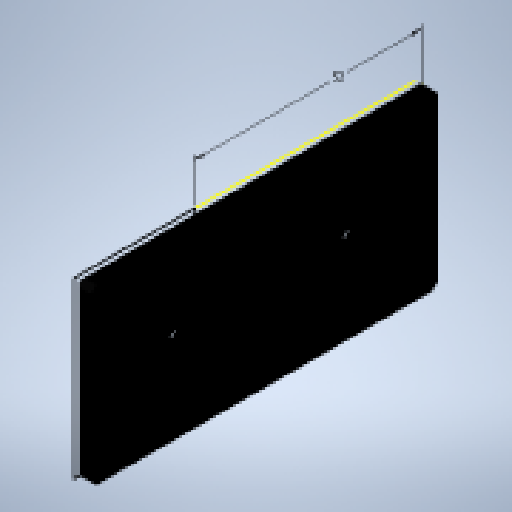
# Autodesk Inventor part: Robotunits CAP_4080_1
Saved by Autodesk Inventor 2023 (Build 270158000, 158)
## iProperties
Category: PARTsolutions
Company: ROBOTUNITS
Created: 2023-08-22
Part Number: Robotunits CAP_4080_1
Material: ABS PlastiK
Catalog Web Link: www.cadenas.de
Description: CAP_1-End Cap
Vendor: ROBOTUNITS
Document SubType Name: Modeling
Designer: psAdmin
Manufacturer: ROBOTUNITS
Mass: 13.3863 g
Surface Area: 73.9102 cm^2
Volume: 12.6286 cm^3
Density: 1.06 g/cm^3
Appearance: Generic
PSOL_IDENT_0: {$CADENAS_DATA/23d-libs/robotunits/pool_bauteile/cap.prj},182 {VTYP=3D},{NB=Robotunits CAP_4080_1},{
PSOL_IDENT_1: LINA=Robotunits CAP_4080_1},{NN=CAP_1},{DATE=24.04.2023 05:54:15},{GEOMDATE=22.02.2023 09:25:00},{VE
PSOL_IDENT_2: RSION=},{LINEID=120},{WBVAR=},{WBNUMERIC=}  {NB=Robotunits CAP_4080_1},{LINA=Robotunits CAP_4080_1},
PSOL_IDENT_3: {KT=DUMMY},{ARTIKEL=CAP_4080},{L=40},{B=80},{H=4},{GEW=0.009},{INFO=INFO},{V=2.000}
NB: Robotunits CAP_4080_1
NN: CAP_1
NT: End Cap
NBSYN: Robotunits $ARTIKEL._1
LINA: Robotunits CAP_4080_1
CATALOG: Robotunits
ARTIKEL: CAP_4080
L: 40
B: 80
H: 4
GEW: 0.009
INFO: INFO
SUPPLIER: ROBOTUNITS
ARTICLENO: Robotunits CAP_4080_1
BOMINFO: Robotunits CAP_4080_1
CREATOR: CADENAS GmbH
Title: Robotunits CAP_4080_1
Author: Cadenas PARTsolutions
Comments: End Cap
Autodesk Inventor part; units mm, degrees
sketch "Skizze_1" plane through (0, 0, 0) normal (1, 0, 0) x (0, 0, -1)
  line L0 (-40, 20) -> (-40, -20)
  line L1 (-40, -20) -> (40, -20)
  line L2 (40, -20) -> (40, 20)
  line L3 (40, 20) -> (-40, 20)
  constraints: 8 end point
extrude "Extrusion1" add sketch "Skizze_1" along normal blind 4
sketch "Sketch2" plane through (0, 0, 0) normal (-1, 0, 0) x (0, 0, 1)
  point P0 (20, 0)
hole "Hole1" at (0, 0, 20) direction (1, 0, 0) diameter 4 depth 4 countersink diameter 8.1 countersink angle 90
sketch "Sketch3" plane through (0, 0, 0) normal (-1, 0, 0) x (0, 0, 1)
  point P0 (-20, 0)
hole "Hole2" at (0, 0, -20) direction (1, 0, 0) diameter 4 depth 4 countersink diameter 8.1 countersink angle 90
ref_plane "CS_ANBAU_CAP_XY" through (0, 0, 0) normal (0, 1, 0) x (1, 0, 0)
ref_plane "CS_ANBAU_CAP_YZ" through (0, 0, 0) normal (1, 0, 0) x (0, 0, -1)
ref_plane "CS_ANBAU_CAP_ZX" through (0, 0, 0) normal (0, 0, -1) x (0, 1, 0)
ref_plane "CS_ANBAU_CAP_90_XY" through (0, 0, 0) normal (0, 0, 1) x (1, 0, 0)
ref_plane "CS_ANBAU_CAP_90_YZ" through (0, 0, 0) normal (1, 0, 0) x (0, 1, 0)
ref_plane "CS_ANBAU_CAP_90_ZX" through (0, 0, 0) normal (0, 1, 0) x (0, 0, 1)
ref_plane "IB_1_XY" through (0, 0, 0) normal (1, 0, 0) x (0, 0, -1)
ref_plane "IB_1_YZ" through (0, 0, 0) normal (0, 0, -1) x (0, 1, 0)
ref_plane "IB_1_ZX" through (0, 0, 0) normal (0, 1, 0) x (1, 0, 0)
ref_plane "IB_10_XY" through (0, -14, 30) normal (1, 0, 0) x (0, 0, -1)
ref_plane "IB_10_YZ" through (0, -14, 30) normal (0, 0, -1) x (0, 1, 0)
ref_plane "IB_10_ZX" through (0, -14, 30) normal (0, 1, 0) x (1, 0, 0)
ref_plane "IB_11_XY" through (0, 14, 30) normal (1, 0, 0) x (0, 0, -1)
ref_plane "IB_11_YZ" through (0, 14, 30) normal (0, 0, -1) x (0, 1, 0)
ref_plane "IB_11_ZX" through (0, 14, 30) normal (0, 1, 0) x (1, 0, 0)
ref_plane "IB_12_XY" through (0, 0, -20) normal (1, 0, 0) x (0, 0, -1)
ref_plane "IB_12_YZ" through (0, 0, -20) normal (0, 0, -1) x (0, 1, 0)
ref_plane "IB_12_ZX" through (0, 0, -20) normal (0, 1, 0) x (1, 0, 0)
ref_plane "IB_2_XY" through (0, 0, -20) normal (1, 0, 0) x (0, 0, -1)
ref_plane "IB_2_YZ" through (0, 0, -20) normal (0, 0, -1) x (0, 1, 0)
ref_plane "IB_2_ZX" through (0, 0, -20) normal (0, 1, 0) x (1, 0, 0)
ref_plane "IB_3_XY" through (0, 0, 20) normal (1, 0, 0) x (0, 0, -1)
ref_plane "IB_3_YZ" through (0, 0, 20) normal (0, 0, -1) x (0, 1, 0)
ref_plane "IB_3_ZX" through (0, 0, 20) normal (0, 1, 0) x (1, 0, 0)
ref_plane "IB_4_XY" through (0, 13.5, -33.5) normal (1, 0, 0) x (0, 0, -1)
ref_plane "IB_4_YZ" through (0, 13.5, -33.5) normal (0, 0, -1) x (0, 1, 0)
ref_plane "IB_4_ZX" through (0, 13.5, -33.5) normal (0, 1, 0) x (1, 0, 0)
ref_plane "IB_5_XY" through (0, 13.5, 33.5) normal (1, 0, 0) x (0, 0, -1)
ref_plane "IB_5_YZ" through (0, 13.5, 33.5) normal (0, 0, -1) x (0, 1, 0)
ref_plane "IB_5_ZX" through (0, 13.5, 33.5) normal (0, 1, 0) x (1, 0, 0)
ref_plane "IB_6_XY" through (0, 1.5, 26.5) normal (1, 0, 0) x (0, 0, -1)
ref_plane "IB_6_YZ" through (0, 1.5, 26.5) normal (0, 0, -1) x (0, 1, 0)
ref_plane "IB_6_ZX" through (0, 1.5, 26.5) normal (0, 1, 0) x (1, 0, 0)
ref_plane "IB_7_XY" through (0, 1.5, -26.5) normal (1, 0, 0) x (0, 0, -1)
ref_plane "IB_7_YZ" through (0, 1.5, -26.5) normal (0, 0, -1) x (0, 1, 0)
ref_plane "IB_7_ZX" through (0, 1.5, -26.5) normal (0, 1, 0) x (1, 0, 0)
ref_plane "IB_8_XY" through (0, -2, 34) normal (1, 0, 0) x (0, 0, -1)
ref_plane "IB_8_YZ" through (0, -2, 34) normal (0, 0, -1) x (0, 1, 0)
ref_plane "IB_8_ZX" through (0, -2, 34) normal (0, 1, 0) x (1, 0, 0)
ref_plane "IB_9_XY" through (0, -2, -34) normal (1, 0, 0) x (0, 0, -1)
ref_plane "IB_9_YZ" through (0, -2, -34) normal (0, 0, -1) x (0, 1, 0)
ref_plane "IB_9_ZX" through (0, -2, -34) normal (0, 1, 0) x (1, 0, 0)
chamfer "Chamfer1" distance 1.25 angle 45 8 edges at (2, -20, 40) (0, -20, 0) (0, 0, 40) (2, -20, -40) (0, 0, -40) (2, 20, -40) (0, 20, 0) (2, 20, 40)
sketch "Sketch5" plane through (4, 0, 0) normal (1, 0, 0) x (0, 0, -1)
  line L0 (-38.75, -20) -> (38.75, -20) projected
  line L1 (-12, -20) -> (-40, -20)
  line L2 (-40, -20) -> (-40, 20)
  line L3 (-40, 20) -> (-12, 20)
  line L4 (-12, 20) -> (-12, -20)
  line L5 (-40, 18.75) -> (-40, -18.75) projected
  line L6 (38.75, 20) -> (-38.75, 20) projected
  line L7 (40, -18.75) -> (40, 18.75) projected
  point P0 (0, 0)
  dimension "d32" = 52
  constraints: 8 end point, 2 collinear, 2 parallel, 1 horizontal, 1 perpendicular, 1 point on line
  measures "d32" distance between parallel lines of L7 L4
extrude "Extrusion2" cut sketch "Sketch5" against normal through all
body "Solid1"
